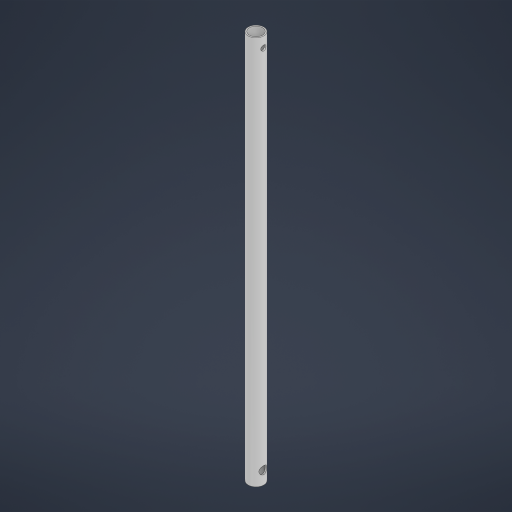
# Autodesk Inventor part: pipe
Saved by Autodesk Inventor 2023 (Build 270158000, 158)
## iProperties
Created: 2022-04-24
Part Number: pipe
Material: Aluminum 6061
Document SubType Name: Modeling
Designer: Norbert Ligas
Density: 2.7 g/cm^3
Appearance: Aluminum - Polished
pipe_length: 300,000 mm
Author: Norbert Ligas
Autodesk Inventor part; units mm, degrees
ref_plane "XZ Plane" through (0, 0, 0) normal (0, 1, 0) x (-1, 0, 0)
ref_plane "XY Plane" through (0, 0, 0) normal (0, 0, 1) x (1, 0, 0)
sketch "Sketch1" plane through (0, 0, 0) normal (0, 1, 0) x (-1, 0, 0)
  circle A0 centre (0, 0) radius 5
  circle A1 centre (0, 0) radius 6
  dimension "d0" = 12
  dimension "d1" = 1
  constraints: 2 centre point, 2 coincident
  measures "d0" diameter of A1
  measures "d1" radial gap between concentric circles of A0 A1
extrude "Extrusion1" add sketch "Sketch1" along normal blind 300
ref_plane "Work Plane3" through (6, 0, 0) normal (1, 0, 0) x (0, 1, 0)
sketch "Sketch2" plane through (6, 0, 0) normal (1, 0, 0) x (0, 1, 0)
  line L0 (0, -6) -> (300, -6) projected
  line L1 (0, 6) -> (300, 6) projected
  line L2 (300, -6) -> (300, 6) projected
  line L3 (-60, 0) -> (360, 0) projected
  point P0 (0, 0)
  point P1 (10, 0)
  point P2 (292, 0)
  point P3 (300, 0)
  dimension "d20" = 10
  dimension "d21" = 8
  constraints: 2 point on line, 1 midpoint
  measures "d20" distance of point (0, 0) point (10, 0)
  measures "d21" distance of point (300, 0) point (292, 0)
hole "Hole1" at (6, 10, 0) direction (-1, 0, 0) diameter 6 end up to face face through (0, 0, 0) facing (0, 1, 0) round with radius 5 far side no
hole "Hole2" at (6, 292, 0) direction (-1, 0, 0) diameter 4 end up to face face through (0, 0, 0) facing (0, 1, 0) round with radius 5 far side no
equation "\"d2\" = pipe_length"
equation "\"pipe_length\" = 300"
body "Solid1"
